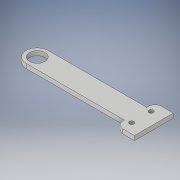
# Autodesk Inventor part: TapeMeasureBracketSide
Saved by Autodesk Inventor 2019 (Build 230136000, 136)
## iProperties
Created: 2018-11-04
Part Number: TapeMeasureBracketSide
Material: Generic
Document SubType Name: Modeling
Designer: mrhftc
Density: 1 g/cm^3
Appearance: Default
Author: mrhftc
Autodesk Inventor part; units mm, degrees
ref_plane "YZ Plane" through (0, 0, 0) normal (1, 0, 0) x (0, 1, 0)
ref_plane "XZ Plane" through (0, 0, 0) normal (0, 1, 0) x (-1, 0, 0)
ref_plane "XY Plane" through (0, 0, 0) normal (0, 0, 1) x (1, 0, 0)
sketch "Main Sketch" plane through (0, 0, 0) normal (0, 1, 0) x (-1, 0, 0)
  line L0 (-57.375, -12.0472) -> (-57.375, 12.0472)
  line L1 (-57.375, 12.0472) -> (47.625, -10) construction
  line L2 (47.625, 10) -> (-57.375, -12.0472) construction
  circle A0 centre (47.625, 0) radius 7
  arc A1 (47.625, -10) -> (47.625, 10) centre (47.625, 0) ccw
  line L3 (-40.875, 17.5) -> (-57.375, 17.5)
  line L4 (-57.375, 17.5) -> (-57.375, -17.5)
  line L5 (-57.375, -17.5) -> (-40.875, -17.5)
  line L6 (-40.875, 17.5) -> (-57.375, -17.5) construction
  line L7 (-57.375, 17.5) -> (-40.875, -17.5) construction
  line L8 (47.625, -10) -> (-40.875, -10)
  line L9 (-40.875, -17.5) -> (-40.875, -10)
  line L10 (-40.875, 10) -> (-40.875, 17.5)
  line L11 (-40.875, 10) -> (47.625, 10)
  point P0 (0, 0)
  point P1 (-49.125, 0)
  dimension "d3" = 14
  dimension "d4" = 105
  dimension "d13" = 16.5
  dimension "d14" = 35
  dimension "d15" = 0
  dimension "d18" = 20
  constraints: 24 end point, 4 parallel, 2 centre point, 2 horizontal, 2 midpoint, 2 point on circle, 2 point on line, 1 coincident, 1 perpendicular
  measures "d3" diameter of A0
  measures "d4" distance from line of L0 A0.centre
  measures "d13" distance of L4.end L5.end
  measures "d14" distance of L3.end L4.end
  measures "d15" distance between parallel lines of L0 L4
  measures "d18" distance between parallel lines of L11 L8
extrude "Main Extrusion" add sketch "Main Sketch" along normal blind 4
sketch "Screw Holes Sketch" plane through (0, 4, 0) normal (0, 1, 0) x (1, 0, 0)
  circle A0 centre (46.125, -8.75) radius 2
  line L0 (57.375, 17.5) -> (40.875, 17.5) projected
  line L1 (40.875, -17.5) -> (57.375, -17.5) projected
  line L2 (35.2664, 0) -> (65.7891, 0)
  line L3 (51.375, -27.0398) -> (51.375, 30.2346) construction
  line L4 (57.375, -17.5) -> (57.375, 17.5) projected
  line L5 (40.875, -10) -> (40.875, -17.5) projected
  circle A1 centre (46.125, 8.75) radius 2
  line L6 (51.375, 27.0398) -> (51.375, -30.2346) construction
  point P0 (0, 0)
  dimension "d21" = 4
  dimension "d22" = 35
  dimension "d23" = 6
  dimension "d24" = 5.25
  dimension "d25" = 5.25
  dimension "d26" = 10.5
  dimension "d27" = 8.75
  dimension "d28" = 17.5
  constraints: 6 end point, 3 symmetric about line, 2 centre point, 1 horizontal, 1 vertical, 1 other
  measures "d21" diameter of A0
  measures "d22" distance between parallel lines of L0 L1
  measures "d23" distance between parallel lines of L4 L3
  measures "d24" distance from line of L3 A0.centre
  measures "d25" distance from line of L5 A0.centre
  measures "d26" distance between parallel lines of L3 L5
  measures "d27" distance from line of L1 A0.centre
  measures "d28" diameter of A0.centre L2
extrude "Screw Holes Cut" cut sketch "Screw Holes Sketch" against normal through all
fillet "Fillet1" radius 6 2 edges at (40.875, 2, -17.5) (40.875, 2, 17.5)
body "Solid3"
